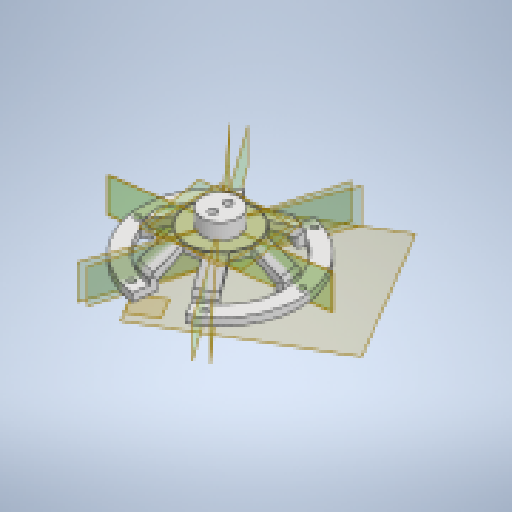
# Autodesk Inventor part: Part3
Saved by Autodesk Inventor 2023.1 (Build 271208000, 208)
## iProperties
Created: 2022-12-25
Part Number: Part3
Material: Generic
Document SubType Name: Modeling
Designer: USER
Density: 1 g/cm^3
Appearance: Default
Author: USER
Autodesk Inventor part; units mm, degrees
ref_plane "YZ Plane" through (0, 0, 0) normal (1, 0, 0) x (0, 1, 0)
ref_plane "XZ Plane" through (0, 0, 0) normal (0, 1, 0) x (-1, 0, 0)
ref_plane "XY Plane" through (0, 0, 0) normal (0, 0, 1) x (1, 0, 0)
ref_plane "Work Plane2" through (19.6864, 42.873, -5.1834) normal (0, 1, 0) x (-0.8594863, 0, 0.5111589)
sketch "Sketch2" plane through (19.6864, 42.873, -5.1834) normal (0, 1, 0) x (-0.8594863, 0, 0.5111589)
  arc A0 (-17.4798, -35.6695) -> (-17.5078, -35.635) centre (19.5623, -5.6019) ccw
  circle A1 centre (19.5623, -5.6019) radius 41.2486
  arc A2 (20.7642, -38.5687) -> (39.4478, 20.7115) centre (19.5697, -5.6078) ccw
  line L0 (44.9118, 27.9461) -> (39.4478, 20.7115)
  line L1 (20.7642, -38.5687) -> (21.0926, -47.6289)
  line L2 (-9.0127, -36.4483) -> (-2.85, -29.7988)
  arc A3 (21.8422, 27.2963) -> (-2.85, -29.7988) centre (19.5697, -5.6078) ccw
  line L3 (21.8422, 27.2963) -> (22.4669, 36.3409)
  circle A4 centre (15.9046, 31.4022) radius 1.65
  circle A5 centre (-15.2782, 9.0389) radius 1.65
  circle A6 centre (-10.0105, -29.5645) radius 1.65
  circle A7 centre (46.7592, 19.795) radius 1.65
  circle A8 centre (54.4084, -19.7505) radius 1.65
  circle A9 centre (26.3689, -42.7588) radius 1.65
  point P0 (22.4122, 35.5482)
  point P1 (-8.4693, -35.862)
  point P2 (21.0634, -46.8231)
  point P3 (44.4299, 27.3079)
  point P4 (21.8422, 27.2963)
  constraints: 10 centre point, 8 end point, 6 point on circle, 1 coincident, 1 other
ref_plane "Work Plane3" through (-0.0004, 59.0758, 0.0003) normal (0, -1, 0) x (0.9884282, 0, -0.1516897)
sketch "Sketch3" plane through (-0.0004, 59.0758, 0.0003) normal (0, -1, 0) x (0.9884282, 0, -0.1516897)
  circle A0 centre (0, 0) radius 16.9271
  circle A1 centre (0, 0) radius 9.6172
  point P0 (0.0005, -0.0002)
  constraints: 2 centre point, 1 coincident
extrude "Extrusion3" add sketch "Sketch3" along normal blind 4
extrude "Extrusion4" add sketch "Sketch2" along normal blind 4 contours A1 L1 A2 L0 | L3 A3 L2 A1
sketch "Sketch4" plane through (19.6864, 46.873, -5.1834) normal (0, 1, 0) x (0.8594863, 0, -0.5111589)
  arc A0 (-21.8422, -27.2963) -> (2.85, 29.7988) centre (-19.5697, 5.6078) ccw projected
  line L0 (8.4693, 35.862) -> (2.85, 29.7988) projected
  arc A1 (-22.4122, -35.5482) -> (8.4693, 35.862) centre (-19.5623, 5.6019) ccw projected
  arc A2 (-20.7642, 38.5687) -> (-39.4478, -20.7115) centre (-19.5697, 5.6078) ccw projected
  line L1 (-20.7642, 38.5687) -> (-21.0634, 46.8231) projected
  line L2 (-44.4299, -27.3079) -> (-39.4478, -20.7115) projected
  arc A3 (-21.0634, 46.8231) -> (-44.4299, -27.3079) centre (-19.5623, 5.6019) ccw projected
  line L3 (-21.8422, -27.2963) -> (-22.4122, -35.5482) projected
  circle A4 centre (-19.5623, 5.6019) radius 29.009
  line L4 (-19.5623, 5.6019) -> (-20.7642, 38.5687)
  line L5 (-19.5623, 5.6019) -> (-30.8338, 36.6073)
  arc A5 (-20.7642, 38.5687) -> (-39.4478, -20.7115) centre (-19.5697, 5.6078) ccw projected
  line L6 (-19.5697, 5.6078) -> (-51.5286, 13.7611)
  line L7 (-19.5697, 5.6078) -> (-47.7825, 22.6925)
  line L8 (-19.5697, 5.6078) -> (-39.4478, -20.7115)
  line L9 (-19.5697, 5.6078) -> (-46.9449, -12.7891)
  line L10 (-21.8422, -27.2963) -> (-19.5697, 5.6078)
  line L11 (-19.5697, 5.6078) -> (-11.6534, -26.4106)
  line L12 (-19.5697, 5.6078) -> (8.6431, -11.4768)
  line L13 (12.5176, -2.0247) -> (-19.5623, 5.6019)
  line L14 (-19.5623, 5.6019) -> (2.85, 29.7988)
  circle A6 centre (-19.5702, 5.6078) radius 9.6172 projected
  line L15 (-19.5702, 5.6078) -> (8.6431, 22.6925)
  point P0 (-19.5697, 5.6078)
  point P1 (-43.6446, -10.5712)
  point P2 (-46.9449, -12.7891)
  point P3 (-37.0532, -17.541)
  point P4 (-44.3756, 20.6294)
  point P5 (-47.7825, 22.6925)
  point P6 (-51.5286, 13.7611)
  point P7 (-47.6701, 12.7768)
  point P8 (-30.8338, 36.6073)
  point P9 (-29.4734, 32.8653)
  point P10 (-20.6192, 34.5916)
  point P11 (5.247, 20.6359)
  point P12 (0.1503, 26.8841)
  point P13 (-12.6053, -22.5606)
  point P14 (-21.5688, -23.3377)
  point P15 (8.6602, -1.1076)
  point P16 (5.2523, -9.4234)
  constraints: 24 end point, 8 point on circle, 1 centre point, 1 coincident, 1 point on line
extrude "Extrusion5" add sketch "Sketch4" along normal blind 4 and the other way blind 4 contours L10 A4 L11 A0 | L12 A4 L13 A0 | L8 A2 L9 A4 | A0 L15 A4 L14 | L6 A2 L7 A4 | A4 L5 A2 L4
ref_plane "Work Plane4" through (0.0164, 42.873, -0.0313) normal (-0.9393098, 0, -0.3430702) x (0, -1, 0)
ref_plane "Work Plane5" through (0.0094, 42.873, 0.0014) normal (0.7457793, 0, -0.666193) x (0, 1, 0)
ref_plane "Work Plane6" through (0.0094, 42.873, 0.0014) normal (-0.7457793, 0, 0.666193) x (0, -1, 0)
ref_plane "Work Plane7" through (0, 42.873, 0) normal (-0.1389368, 0, -0.9903012) x (0, 1, 0)
ref_plane "Work Plane9" through (0, 42.873, 0) normal (-0.8119888, 0, 0.583673) x (0, 1, 0)
ref_plane "Work Plane10" through (0.0135, 42.873, 0.0001) normal (-0.1470463, 0, -0.9891296) x (0, -1, 0)
ref_plane "Work Plane11" through (0, 42.873, 0) normal (-0.9620321, 0, -0.2729362) x (0, 1, 0)
ref_plane "Work Plane12" through (19.6864, 33.4105, -5.1834) normal (0, 1, 0) x (0.8594863, 0, -0.5111589)
sketch "Sketch7" plane through (19.6864, 33.4105, -5.1834) normal (0, 1, 0) x (0.8594863, 0, -0.5111589)
  line L0 (-20.7642, 38.5687) -> (-20.6192, 34.5916) projected
  line L1 (-20.6321, 34.9451) -> (-29.5995, 33.2121)
  line L2 (-29.4734, 32.8653) -> (-30.8338, 36.6073) projected
  point P0 (-19.5697, 5.6078)
  constraints: 2 end point, 2 point on line
sketch "Sketch9" plane through (19.6864, 50.873, -5.1834) normal (0, 1, 0) x (0.8594863, 0, -0.5111589)
  circle A0 centre (-19.5697, 5.6078) radius 32.9825
  constraints: 1 centre point, 1 coincident
extrude "Extrusion7" cut sketch "Sketch9" against normal blind 5.5875 draft -50
ref_plane "Work Plane13" through (-0.0004, 59.0658, 0.0003) normal (0, 1, 0) x (1, 0, 0)
sketch "Sketch10" plane through (-0.0004, 59.0658, 0.0003) normal (0, 1, 0) x (1, 0, 0)
  line L0 (16.3511, 7.568) -> (17.9444, -1.6213)
  line L1 (17.9444, -1.6213) -> (14.7296, -10.376)
  line L2 (14.7296, -10.376) -> (7.5681, -16.3504)
  line L3 (7.5681, -16.3504) -> (-1.6211, -17.9437)
  line L4 (-1.6211, -17.9437) -> (-10.3758, -14.7289)
  line L5 (-10.3758, -14.7289) -> (-16.3502, -7.5675)
  line L6 (-16.3502, -7.5675) -> (-17.9435, 1.6218)
  line L7 (-17.9435, 1.6218) -> (-14.7287, 10.3765)
  line L8 (-14.7287, 10.3765) -> (-7.5673, 16.3509)
  line L9 (-7.5673, 16.3509) -> (1.6219, 17.9442)
  line L10 (1.6219, 17.9442) -> (10.3767, 14.7294)
  line L11 (10.3767, 14.7294) -> (16.3511, 7.568)
  circle A0 centre (0, 0) radius 16.9271 projected
  circle A1 centre (0, 0) radius 9.6172
  point P0 (0.0004, 0.0003)
  point P1 (0.0004, 0.0003)
  constraints: 24 end point, 2 coincident, 1 centre point, 25 other
extrude "Extrusion8" add sketch "Sketch10" against normal blind 4 contours L0 L1 L2 L3 L4 L5 L6 L7 L8 L9 L10 L11
loft "Loft2" add section 1 edges at (-5.9989, 59.0658, 16.3366) (-10.3762, 57.0658, 14.7292) (-5.9989, 55.0658, 16.3366) (-1.6215, 57.0658, 17.944) section 2 edges at (-13.2734, 49.2047, 28.0084) (-9.0021, 50.873, 31.7303) (-3.4129, 49.2061, 30.8075) (-7.9172, 47.5378, 27.9065)
loft "Loft3" add section 1 edges at (-30.9901, 49.202, -0.2469) (-32.6626, 50.873, 4.5825) (-29.7261, 49.2023, 8.7653) (-28.7186, 47.5312, 4.0292) section 2 edges at (-17.1473, 59.0658, 2.9731) (-17.944, 57.0658, -1.6215) (-17.1473, 55.0658, 2.9731) (-16.3507, 57.0658, 7.5677)
loft "Loft4" add section 1 edges at (-11.1484, 59.0658, -13.3635) (-7.5677, 57.0658, -16.3507) (-11.1484, 55.0658, -13.3635) (-14.7292, 57.0658, -10.3762) section 2 edges at (-16.7615, 49.1496, -25.993) (-21.9682, 50.873, -24.6017) (-23.9364, 49.1488, -19.5849) (-19.3162, 47.5327, -21.633)
loft "Loft5" add section 1 edges at (14.5518, 49.1539, -27.2973) (11.3197, 50.873, -30.9792) (6.4755, 49.1527, -30.247) (9.9572, 47.5405, -27.2487) section 2 edges at (5.9989, 59.0658, -16.3366) (10.3762, 57.0658, -14.7292) (5.9989, 55.0658, -16.3366) (1.6215, 57.0658, -17.944)
loft "Loft6" add section 1 edges at (17.1473, 59.0658, -2.9731) (17.944, 57.0658, 1.6215) (17.1473, 55.0658, -2.9731) (16.3507, 57.0658, -7.5677) section 2 edges at (30.9995, 49.2099, 0.247) (32.6243, 50.873, -4.8479) (29.5274, 49.1563, -9.2309) (28.703, 47.5465, -4.2649)
loft "Loft7" add section 1 edges at (11.1484, 59.0658, 13.3635) (7.5677, 57.0658, 16.3507) (11.1484, 55.0658, 13.3635) (14.7292, 57.0658, 10.3762) section 2 edges at (13.9718, 49.2082, 27.6712) (19.251, 50.873, 26.7814) (21.7774, 49.2091, 22.0617) (16.9357, 47.5444, 23.5603)
fillet "Fillet1" radius 3 6 edges at (19.251, 50.873, 26.7814) (32.6243, 50.873, -4.8479) (11.3197, 50.873, -30.9792) (-21.9682, 50.873, -24.6017) (-32.6626, 50.873, 4.5825) (-9.0021, 50.873, 31.7303)
extrude "Extrusion9" add sketch "Sketch10" along normal blind 8.2 and the other way blind 4 contours A1
sketch "Sketch11" plane through (-0.0004, 67.2658, 0.0003) normal (0, 1, 0) x (1, 0, 0)
  circle A0 centre (0.0004, 4.036) radius 2.1
  circle A1 centre (0.0004, -3.8664) radius 2.1
  point P0 (0.0004, 0.0003)
  dimension "d70" = 4.2
  dimension "d71" = 4.2
  constraints: 2 centre point
  measures "d70" diameter of A0
  measures "d71" diameter of A1
extrude "Extrusion10" cut sketch "Sketch11" against normal blind 8.2
body "Solid2"
